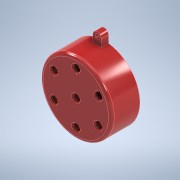
# Autodesk Inventor part: Conector2
Saved by Autodesk Inventor 2021 (Build 250183000, 183)
## iProperties
Created: 2021-05-27
Part Number: Conector2
Material: Genérico
Document SubType Name: Modeling
Designer: rubia
Density: 1 g/cm^3
Appearance: Vermelho
GlobalPropertyList: <PropertyList/>
Author: rubia
Autodesk Inventor part; units mm, degrees
ref_plane "YZ Plane" through (0, 0, 0) normal (1, 0, 0) x (0, 1, 0)
ref_plane "XZ Plane" through (0, 0, 0) normal (0, 1, 0) x (-1, 0, 0)
ref_plane "XY Plane" through (0, 0, 0) normal (0, 0, 1) x (1, 0, 0)
sketch "Esboço1" plane through (0, 0, 0) normal (0, 0, 1) x (1, 0, 0)
  circle A0 centre (0, 0) radius 25
  dimension "d0" = 50
  constraints: 1 centre point, 1 coincident
  measures "d0" diameter of A0
extrude "Extrusão1" add sketch "Esboço1" along normal blind 20
fillet "Arredondamento1" radius 2 1 edges at (-25, 0, 20)
sketch "Esboço2" plane through (0, 0, 20) normal (0, 0, 1) x (1, 0, 0)
  circle A0 centre (0, 0) radius 2.5
  circle A1 centre (0, 18) radius 2.5
  dimension "d4" = 5
  dimension "d5" = 5
  dimension "d6" = 18
  constraints: 2 centre point, 1 coincident
  measures "d4" diameter of A0
  measures "d5" diameter of A1
  measures "d6" distance of point (0, 0) A1.centre
extrude "Extrusão2" cut sketch "Esboço2" against normal blind 15
chamfer "Chanfro1" distance 0.6 angle 45 2 edges at (-2.5, 0, 20) (-2.5, 18, 20)
pattern_circular "Padrão circular1" count 6 over 360 about axis through (0, 0, 0) along (0, 0, 1) of "Extrusão2", "Chanfro1"
sketch "Esboço3" plane through (0, 0, 0) normal (0, 0, -1) x (-1, 0, 0)
  arc A0 (3, 30) -> (-3, 30) centre (0, 30) ccw
  circle A1 centre (0, 30) radius 1.5
  line L0 (3, 30) -> (3, 24.3841)
  line L1 (-3, 30) -> (-3, 24.3841)
  line L2 (-3, 24.3841) -> (3, 24.3841)
  point P0 (0, 0)
  dimension "d15" = 6
  dimension "d16" = 3
  dimension "d17" = 30
  constraints: 6 end point, 2 centre point, 2 point on circle, 2 vertical, 1 coincident, 1 horizontal, 1 tangent
  measures "d15" diameter of A0
  measures "d16" diameter of A1
  measures "d17" distance of point (0, 0) A0.centre
extrude "Extrusão3" add sketch "Esboço3" against normal blind 5
mirror "Espelhamento1" about plane through (0, 0, 0) normal (0, 1, 0) of "Extrusão3"
sketch "Esboço4" plane through (0, 0, 20) normal (0, 0, 1) x (1, 0, 0)
  circle A0 centre (0, 0) radius 3.1 projected
sketch "Esboço5" plane through (0, 0, 20) normal (0, 0, 1) x (1, 0, 0)
  circle A0 centre (0, 18) radius 3.1 projected
sketch "Esboço6" plane through (0, 0, 20) normal (0, 0, 1) x (1, 0, 0)
  circle A0 centre (15.5885, 9) radius 3.1 projected
sketch "Esboço7" plane through (0, 0, 20) normal (0, 0, 1) x (1, 0, 0)
  circle A0 centre (15.5885, -9) radius 3.1 projected
sketch "Esboço8" plane through (0, 0, 20) normal (0, 0, 1) x (1, 0, 0)
  circle A0 centre (0, -18) radius 3.1 projected
sketch "Esboço9" plane through (0, 0, 20) normal (0, 0, 1) x (1, 0, 0)
  circle A0 centre (-15.5885, -9) radius 3.1 projected
sketch "Esboço10" plane through (0, 0, 20) normal (0, 0, 1) x (1, 0, 0)
  circle A0 centre (-15.5885, 9) radius 3.1 projected
